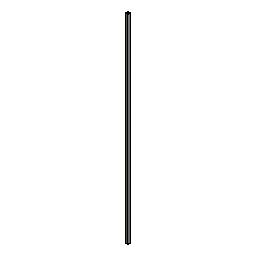
cf_rod_45 (Autodesk Fusion 360 design; units mm, degrees)
Autodesk Fusion 360 part; units mm, degrees
sketch "Sketch1" plane through (0, 0, 0) normal (0, 1, 0) x (1, 0, 0)
  line L0 (0, 0) -> (6, 0)
  line L1 (6, 0) -> (6, -6)
  line L2 (6, -6) -> (0, -6)
  line L3 (0, -6) -> (0, 0)
  line L4 (5, -5) -> (1, -5)
  line L5 (1, -5) -> (1, -1)
  line L6 (1, -1) -> (5, -1)
  line L7 (5, -1) -> (5, -5)
  dimension "d1" = 6
  dimension "d2" = 6
  dimension "d3" = 1
  constraint horizontal L0
  constraint vertical L1
  constraint horizontal L2
  constraint vertical L3
  constraint coincident L0.start L3.end
  measures "d1" distance of L0.start L0.end
  measures "d2" distance of L0.start L2.end
extrude "Extrude1" add sketch "Sketch1" along normal blind 450
